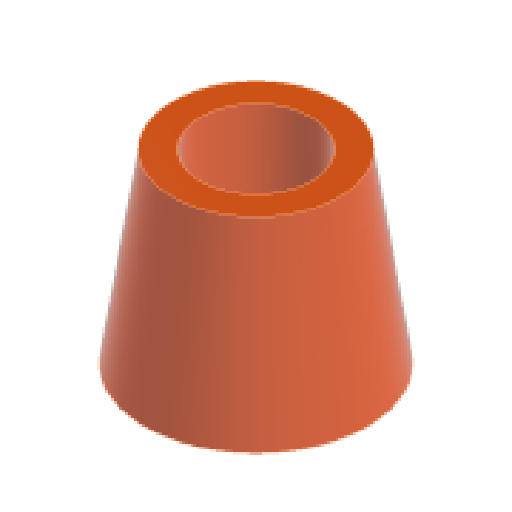
# Autodesk Inventor part: Idler Spacer
Saved by Autodesk Inventor 2023.2 (Build 272271000, 271)
## iProperties
Created: 2023-02-04
Part Number: Idler Spacer
Material: ABS Plastic
Document SubType Name: Modeling
Designer: remop
Density: 1.06 g/cm^3
Appearance: Smooth - Light Orange
Author: remop
Autodesk Inventor part; units mm, degrees
ref_plane "YZ Plane" through (0, 0, 0) normal (1, 0, 0) x (0, 1, 0)
ref_plane "XZ Plane" through (0, 0, 0) normal (0, 1, 0) x (-1, 0, 0)
ref_plane "XY Plane" through (0, 0, 0) normal (0, 0, 1) x (1, 0, 0)
sketch "Sketch1" plane through (0, 0, 0) normal (0, 0, 1) x (1, 0, 0)
  line L0 (0, 0) -> (0, 10)
  line L1 (3, 0) -> (3, 10)
  line L2 (3, 0) -> (6, 0)
  line L3 (6, 0) -> (4.5, 10)
  line L4 (4.5, 10) -> (3, 10)
  dimension "d0" = 10
  dimension "d1" = 6
  dimension "d2" = 12
  dimension "d3" = 9
  constraints: 10 end point, 2 horizontal alignment, 2 vertical, 1 horizontal, 1 parallel
  measures "d0" distance of L1.start L1.end
  measures "d1" diameter of L1 L0
  measures "d2" diameter of L2.end L0
  measures "d3" diameter of L3.end L0
revolve "Revolution1" add sketch "Sketch1" angle 360 about axis through (0, 0, 0) along (0, 1, 0)
body "Solid1"
